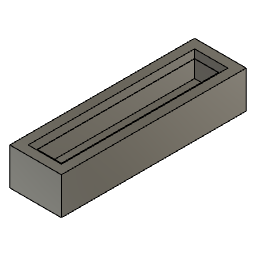
basic_piano_key_mold (Autodesk Fusion 360 design; units mm, degrees)
Autodesk Fusion 360 part; units mm, degrees
sketch "Sketch1" plane through (0, 0, 0) normal (0, 0, 1) x (1, 0, 0)
  line L0 (0, 0) -> (39.4, 0)
  line L1 (39.4, 0) -> (39.4, 141)
  line L2 (39.4, 141) -> (0, 141)
  line L3 (0, 141) -> (0, 0)
  line L4 (7, 7) -> (32.4, 7)
  line L5 (32.4, 7) -> (32.4, 134)
  line L6 (32.4, 134) -> (7, 134)
  line L7 (7, 134) -> (7, 7)
  line L8 (10, 10) -> (29.4, 10)
  line L9 (29.4, 10) -> (29.4, 131)
  line L10 (29.4, 131) -> (10, 131)
  line L11 (10, 131) -> (10, 10)
  line L12 (11, 11) -> (28.4, 11)
  line L13 (28.4, 11) -> (28.4, 130)
  line L14 (28.4, 130) -> (11, 130)
  line L15 (11, 130) -> (11, 11)
  dimension "d1" = 39.4
  dimension "d2" = 141
  dimension "d3" = 25.4
  dimension "d4" = 127
  dimension "d5" = 7
  dimension "d6" = 7
  dimension "d7" = 19.4
  dimension "d8" = 121
  dimension "d9" = 3
  dimension "d10" = 3
  dimension "d11" = 17.4
  dimension "d12" = 119
  dimension "d13" = 1
  dimension "d14" = 1
  constraint horizontal L0
  constraint vertical L1
  constraint horizontal L2
  constraint vertical L3
  constraint coincident L0.start L3.end
  constraint horizontal L4
  constraint vertical L5
  constraint horizontal L6
  constraint vertical L7
  constraint horizontal L8
  constraint vertical L9
  constraint horizontal L10
  constraint vertical L11
  constraint horizontal L12
  constraint vertical L13
  constraint horizontal L14
  constraint vertical L15
  measures "d1" distance of L0.start L0.end
  measures "d2" distance of L0.start L2.end
  measures "d3" distance of L4.start L4.end
  measures "d4" distance of L4.start L6.end
  measures "d5" distance of L3 L7
  measures "d6" distance of L0 L4
  measures "d7" distance of L8.start L8.end
  measures "d8" distance of L8.start L10.end
  measures "d9" distance of L7 L11
  measures "d10" distance of L4 L8
  measures "d11" distance of L12.start L12.end
  measures "d12" distance of L12.start L14.end
  measures "d13" distance of L11 L15
  measures "d14" distance of L10 L14
extrude "Extrude1" add sketch "Sketch1" along normal blind 1 contours L0 L1 L2 L3 | L4 L5 L6 L7 | L8 L9 L10 L11 | L12 L13 L14 L15
sketch "Sketch2" plane through (0, 0, 1) normal (0, 0, 1) x (-1, 0, 0)
  line L0 (0, -141) -> (0, 0)
  line L1 (0, 0) -> (-39.4, 0)
  line L2 (-39.4, 0) -> (-39.4, -141)
  line L3 (-39.4, -141) -> (0, -141)
  line L4 (-7, -7) -> (-32.4, -7)
  line L5 (-32.4, -7) -> (-32.4, -134)
  line L6 (-32.4, -134) -> (-7, -134)
  line L7 (-7, -134) -> (-7, -7)
  line L8 (-10, -10) -> (-29.4, -10)
  line L9 (-29.4, -10) -> (-29.4, -131)
  line L10 (-29.4, -131) -> (-10, -131)
  line L11 (-10, -131) -> (-10, -10)
  line L12 (-11, -11) -> (-28.4, -11)
  line L13 (-28.4, -11) -> (-28.4, -130)
  line L14 (-28.4, -130) -> (-11, -130)
  line L15 (-11, -130) -> (-11, -11)
  dimension "d17" = 25.4
  dimension "d18" = 127
  dimension "d19" = 19.4
  dimension "d20" = 121
  dimension "d21" = 17.4
  dimension "d22" = 119
  dimension "d23" = 7
  dimension "d24" = 7
  dimension "d25" = 3
  dimension "d26" = 3
  dimension "d27" = 1
  dimension "d28" = 1
  constraint horizontal L4
  constraint vertical L5
  constraint horizontal L6
  constraint vertical L7
  constraint horizontal L8
  constraint vertical L9
  constraint horizontal L10
  constraint vertical L11
  constraint horizontal L12
  constraint vertical L13
  constraint horizontal L14
  constraint vertical L15
  measures "d17" distance of L4.start L4.end
  measures "d18" distance of L4.start L6.end
  measures "d19" distance of L8.start L8.end
  measures "d20" distance of L8.start L10.end
  measures "d21" distance of L12.start L12.end
  measures "d22" distance of L12.start L14.end
  measures "d23" distance of L0 L7
  measures "d24" distance of L1 L4
  measures "d25" distance of L7 L11
  measures "d26" distance of L4 L8
  measures "d27" distance of L11 L15
  measures "d28" distance of L8 L12
extrude "Extrude2" add sketch "Sketch2" along normal blind 12 draft -1 contours L12 L13 L14 L15
sketch "Sketch3" plane through (0, 0, 1) normal (0, 0, 1) x (-1, 0, 0)
  line L0 (-11, -130) -> (-28.4, -130)
  line L1 (-28.4, -130) -> (-28.4, -11)
  line L2 (-28.4, -11) -> (-11, -11)
  line L3 (-11, -11) -> (-11, -130)
  line L4 (0, -141) -> (0, 0)
  line L5 (0, 0) -> (-39.4, 0)
  line L6 (-39.4, 0) -> (-39.4, -141)
  line L7 (-39.4, -141) -> (0, -141)
  line L8 (-7, -7) -> (-32.4, -7)
  line L9 (-32.4, -7) -> (-32.4, -134)
  line L10 (-32.4, -134) -> (-7, -134)
  line L11 (-7, -134) -> (-7, -7)
  dimension "d31" = 25.4
  dimension "d32" = 127
  dimension "d33" = 7
  dimension "d34" = 7
  constraint horizontal L8
  constraint vertical L9
  constraint horizontal L10
  constraint vertical L11
  measures "d31" distance of L8.start L8.end
  measures "d32" distance of L8.start L10.end
  measures "d33" distance of L4 L11
  measures "d34" distance of L5 L8
extrude "Extrude3" add sketch "Sketch3" along normal blind 25.4 contours L4 L5 L6 L7
sketch "Sketch4" plane through (0, 0, 1) normal (0, 0, 1) x (-1, 0, 0)
  line L0 (-7, -7) -> (-32.4, -7)
  line L1 (-32.4, -7) -> (-32.4, -134)
  line L2 (-32.4, -134) -> (-7, -134)
  line L3 (-7, -134) -> (-7, -7)
  line L4 (-11, -130) -> (-28.4, -130)
  line L5 (-28.4, -130) -> (-28.4, -11)
  line L6 (-28.4, -11) -> (-11, -11)
  line L7 (-11, -11) -> (-11, -130)
  line L8 (-10, -10) -> (-29.4, -10)
  line L9 (-29.4, -10) -> (-29.4, -131)
  line L10 (-29.4, -131) -> (-10, -131)
  line L11 (-10, -131) -> (-10, -10)
  dimension "d37" = 19.4
  dimension "d38" = 121
  dimension "d39" = 3
  dimension "d40" = 3
  constraint horizontal L8
  constraint vertical L9
  constraint horizontal L10
  constraint vertical L11
  measures "d37" distance of L8.start L8.end
  measures "d38" distance of L8.start L10.end
  measures "d39" distance of L3 L11
  measures "d40" distance of L0 L8
extrude "Extrude4" add sketch "Sketch4" along normal blind 24.4 draft -1 contours L8 L9 L10 L11
extrude "Extrude5" add 1 faces at (2.3333, 49.3333, 26.4) along direction (0, 0, 1) blind 2
